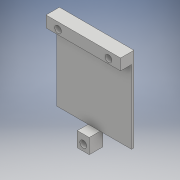
# Autodesk Inventor part: imu_bottom_cover
Saved by Autodesk Inventor 2018 (Build 220112000, 112)
## iProperties
Created: 2020-02-18
Part Number: imu_bottom_cover
Material: Generic
Document SubType Name: Modeling
Designer: bitbots
Density: 1 g/cm^3
Appearance: Default
Author: bitbots
Autodesk Inventor part; units mm, degrees
ref_plane "YZ Plane" through (0, 0, 0) normal (1, 0, 0) x (0, 1, 0)
ref_plane "XZ Plane" through (0, 0, 0) normal (0, 1, 0) x (-1, 0, 0)
ref_plane "XY Plane" through (0, 0, 0) normal (0, 0, 1) x (1, 0, 0)
sketch "Sketch1" plane through (0, 0, 0) normal (0, 1, 0) x (-1, 0, 0)
  line L0 (-15, 20) -> (15, 20)
  line L1 (15, 20) -> (15, -20)
  line L2 (15, -20) -> (-15, -20)
  line L3 (-15, -20) -> (-15, 20)
  line L4 (-15, 20) -> (15, -20) construction
  line L5 (15, 20) -> (-15, -20) construction
  point P0 (0, 0)
  dimension "d0" = 30
  dimension "d1" = 40
  constraints: 12 end point, 2 midpoint, 2 parallel, 1 horizontal, 1 perpendicular
  measures "d0" distance of L1.end L2.end
  measures "d1" distance of L0.end L1.end
extrude "Extrusion1" add sketch "Sketch1" along normal blind 1
sketch "Sketch3" plane through (0, 1, 0) normal (0, 1, 0) x (1, 0, 0)
  line L0 (15, 20) -> (-15, 20) projected
  line L1 (-15, 20) -> (-2.4, 20)
  line L2 (-2.4, 20) -> (-2.4, 14)
  line L3 (-2.4, 14) -> (-15, 14)
  line L4 (-15, 14) -> (-15, 20)
  line L5 (0, 0) -> (0, 20) construction
  line L6 (15, 20) -> (2.4, 20)
  line L7 (2.4, 20) -> (2.4, 14)
  line L8 (2.4, 14) -> (15, 14)
  line L9 (15, 14) -> (15, 20)
  dimension "d7" = 12.6
  dimension "d8" = 6
  dimension "d9" = 12.6
  dimension "d10" = 6
  constraints: 18 end point, 4 parallel, 2 horizontal, 2 perpendicular, 1 midpoint
  measures "d7" distance of L2.end L3.end
  measures "d8" distance between parallel lines of L0 L3
  measures "d9" distance of L8.end L7.end
  measures "d10" distance of L7.end L6.end
extrude "Extrusion3" cut sketch "Sketch3" against normal up to surface (1 mm away)
sketch "Sketch8" plane through (0, 0, 0) normal (0, -1, 0) x (1, 0, 0)
  line L0 (2.4, -20) -> (-2.4, -20) projected
  line L1 (2.4, -20) -> (0, -20)
  line L2 (0, -20) -> (0, -17.5)
  line L3 (-2.4, -20) -> (-2.4, -14) projected
  line L4 (2.4, -20) -> (-2.4, -20)
  line L5 (-2.4, -20) -> (-2.4, -14)
  line L6 (-2.4, -14) -> (2.4, -14)
  line L7 (2.4, -14) -> (2.4, -20)
  line L8 (-15, 20) -> (15, 20) projected
  line L9 (15, 20) -> (10.15, 20)
  line L10 (15, 20) -> (19.85, 20) construction
  line L11 (10.15, 20) -> (10.15, 17.4)
  line L12 (10.15, 17.4) -> (-10.15, 17.4)
  line L13 (10.15, 17.4) -> (30.45, 17.4) construction
  circle A0 centre (-10.15, 17.4) radius 1.35
  circle A1 centre (10.15, 17.4) radius 1.35
  line L14 (15, 20) -> (15, -14) projected
  line L15 (15, 20) -> (-15, 20)
  line L16 (-15, 20) -> (-15, 15.5)
  line L17 (-15, 15.5) -> (15, 15.5)
  line L18 (15, 15.5) -> (15, 20)
  circle A2 centre (0, -17.5) radius 1.35
  point P0 (0, 0)
  dimension "d34" = 2.5
  dimension "d35" = 4.85
  dimension "d36" = 180
  dimension "d39" = 2.6
  dimension "d40" = 20.3
  dimension "d41" = 180
  dimension "d42" = 2.7
  dimension "d43" = 2.7
  dimension "d44" = 30
  dimension "d45" = 4.5
  dimension "d46" = 2.7
  constraints: 30 end point, 5 horizontal, 4 parallel, 3 centre point, 3 coincident, 3 collinear, 3 perpendicular, 1 midpoint, 1 vertical
  measures "d34" distance of L1.end L2.end
  measures "d35" distance of L8.end L9.end
  measures "d36" angle of L9 L10
  measures "d39" distance of L9.end L11.end
  measures "d40" distance of L11.end L12.end
  measures "d41" angle of L12 L13
  measures "d42" diameter of A0
  measures "d43" diameter of A1
  measures "d44" distance of L17.end L16.end
  measures "d45" distance of L16.end L15.end
  measures "d46" diameter of A2
extrude "Extrusion7" add sketch "Sketch8" along normal blind 4.4
sketch "Sketch9" plane through (0, 0, 0) normal (0, -1, 0) x (1, 0, 0)
  circle A0 centre (10.15, 17.4) radius 1.35 projected
  circle A1 centre (-10.15, 17.4) radius 1.35 projected
  circle A2 centre (0, -17.5) radius 1.35 projected
  point P0 (0, 0)
extrude "Extrusion8" cut sketch "Sketch9" against normal up to surface (1 mm away)
body "Solid1"
